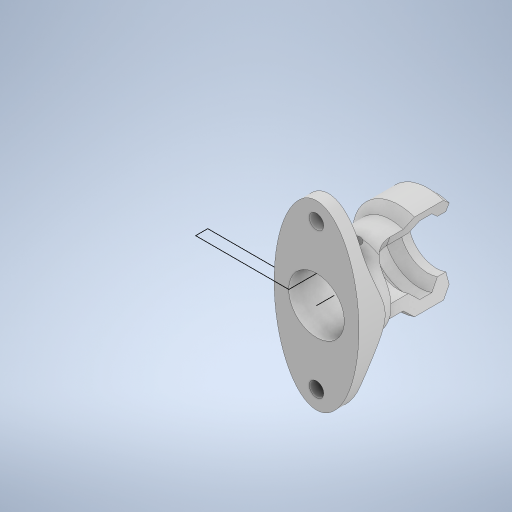
# Autodesk Inventor part: scan lens
Saved by Autodesk Inventor 2024 (Build 280153000, 153)
## iProperties
Created: 2025-02-23
Part Number: scan lens
Material: Generic
Document SubType Name: Modeling
Designer: Williamow
Density: 1 g/cm^3
Appearance: Default
Author: Williamow
Autodesk Inventor part; units mm, degrees
ref_plane "YZ Plane" through (0, 0, 0) normal (1, 0, 0) x (0, 1, 0)
ref_plane "XZ Plane" through (0, 0, 0) normal (0, 1, 0) x (-1, 0, 0)
ref_plane "XY Plane" through (0, 0, 0) normal (0, 0, 1) x (1, 0, 0)
sketch "Sketch1" plane through (0, 0, 0) normal (0, 1, 0) x (-1, 0, 0)
  line L0 (0, 0) -> (0, -1.4662)
  line L1 (2.3, 0) -> (10, 0)
  line L2 (10, 0) -> (10, -1)
  line L3 (10, -1) -> (3.1, -1)
  line L4 (3.1, -1) -> (3.1, -6.1)
  line L5 (3.1, -6.1) -> (3.8, -6.8)
  line L6 (3.8, -6.8) -> (3.8, -9.2)
  line L7 (3.8, -9.2) -> (3.1, -9.9)
  line L8 (3.1, -9.9) -> (2.3, -9.9)
  line L9 (2.3, -9.9) -> (2.3, -9.2)
  line L10 (2.3, -9.2) -> (3, -8.5)
  line L11 (3, -8.5) -> (3, -7.5)
  line L12 (3, -7.5) -> (2.3, -6.8)
  line L13 (2.3, -6.8) -> (2.3, 0)
  line L14 (2.3, -3) -> (3.1, -3)
  circle A0 centre (0, -3) radius 0.6
  point P0 (3, -8)
  dimension "d0" = 1
  dimension "d1" = 1
  dimension "d2" = 0.8
  dimension "d3" = 0.8
  dimension "d4" = 0.7
  dimension "d5" = 3
  dimension "d6" = 10
  dimension "d7" = 8
  dimension "d8" = 3
  dimension "d21" = 1.2
  dimension "d24" = 2.3
  constraints: 30 end point, 7 perpendicular, 5 parallel, 4 horizontal alignment, 4 point on line, 2 vertical, 1 centre point, 1 horizontal, 1 midpoint, 1 vertical alignment
  measures "d0" distance of L1.end L2.end
  measures "d1" distance of L10.end L11.end
  measures "d2" distance of L7.end L8.end
  measures "d3" distance between parallel lines of L6 L11
  measures "d4" distance from line of L9.end L11
  measures "d5" horizontal distance of L0.start point (3, -8)
  measures "d6" distance of L0.start L1.end
  measures "d7" vertical distance of L0.start point (3, -8)
  measures "d8" distance between parallel lines of L1 L14
  measures "d21" diameter of A0
  measures "d24" distance of L0.start L1.start
revolve "Revolution1" add sketch "Sketch1" angle 220 mid plane about axis through (0, 0, 0) along (0, 0, -1) contours L14 L4 L5 L6 L7 L8 L9 L10 L11 L12 L13
revolve "Revolution2" add sketch "Sketch1" angle 360 about axis through (0, 0, 0) along (0, 0, -1) contours L1 L2 L3 L4 L14 L13
sketch "Sketch2" plane through (0, 0, 0) normal (0, 0, 1) x (1, 0, 0)
  circle A0 centre (0, 6) radius 0.6
  circle A1 centre (0, -6) radius 0.6
  ellipse E0 centre (0, 0) end of major axis (0, -7.5) minor radius 3.5
  circle A2 centre (0, 0) radius 10 projected
  dimension "d13" = 3.5
  dimension "d14" = 7.5
  dimension "d11" = 1.2
  dimension "d12" = 6
  dimension "d18" = 6
  dimension "d19" = 6
  constraints: 2 centre point, 2 coincident, 1 equal radius, 1 vertical alignment, 2 other
  measures "d11" diameter of A0
  measures "d12" distance of A0.centre point (0, 0)
  measures "d18" distance of point (0, 0) A0.centre
  measures "d19" distance of A1.centre point (0, 0)
extrude "Extrusion1" cut sketch "Sketch2" against normal blind 2
fillet "Fillet1" radius 2.54 1 edges at (3.1, 0, -1)
fillet "Fillet2" radius 2 2 edges at (0.9334, 2.5645, -3) (0.9334, -2.5645, -3)
extrude "Extrusion2" cut sketch "Sketch1" along normal blind 25.4 contours A0
body "Solid1"
